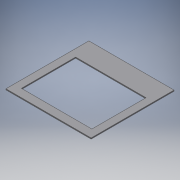
# Autodesk Inventor part: Frontpanel
Saved by Autodesk Inventor 2016 (Build 200138000, 138)
## iProperties
Created: 2018-06-19
Part Number: Frontpanel
Material: Generic
Document SubType Name: Modeling
Designer: suku
Density: 1 g/cm^3
Appearance: Default
Author: suku
Autodesk Inventor part; units mm, degrees
ref_plane "YZ Plane" through (0, 0, 0) normal (1, 0, 0) x (0, 1, 0)
ref_plane "XZ Plane" through (0, 0, 0) normal (0, 1, 0) x (-1, 0, 0)
ref_plane "XY Plane" through (0, 0, 0) normal (0, 0, 1) x (1, 0, 0)
sketch "Sketch1" plane through (0, 0, 0) normal (0, 0, 1) x (1, 0, 0)
  line L0 (109.2, 0) -> (109.2, -84) projected
  line L1 (0, -84) -> (0, 0) projected
  line L2 (0, -84) -> (109.2, -84)
  line L3 (109.2, -84) -> (109.2, 0)
  line L4 (109.2, 0) -> (0, 0)
  line L5 (0, 0) -> (0, -84)
  line L6 (-11.4, 31.9489) -> (120.6, 31.9489)
  line L7 (120.6, 31.9489) -> (120.6, -96.5511)
  line L8 (120.6, -96.5511) -> (-11.4, -96.5511)
  line L9 (-11.4, -96.5511) -> (-11.4, 31.9489)
  line L10 (117.1, 20.1989) -> (-7.9, 20.1989)
  line L11 (-7.9, 20.1989) -> (-7.9, -84.8011)
  line L12 (-7.9, -84.8011) -> (117.1, -84.8011)
  line L13 (117.1, -84.8011) -> (117.1, 20.1989)
  line L14 (-7.9, -84.8011) -> (-7.9, -96.5511)
  line L15 (-7.9, 20.1989) -> (-7.9, 31.9489)
  line L16 (109.2, -42) -> (117.1, -42)
  line L17 (0, -42) -> (-7.9, -42)
  line L18 (120.6, -32.3011) -> (117.1, -32.3011)
  line L19 (-7.9, -32.3011) -> (-11.4, -32.3011)
  dimension "d0" = 128.5
  dimension "d1" = 105
  dimension "d3" = 125
  dimension "d4" = 132
  constraints: 36 end point, 6 midpoint, 6 parallel, 6 point on line, 5 perpendicular, 3 collinear, 3 horizontal
  measures "d0" distance between parallel lines of L8 L6
  measures "d1" distance of L10.end L11.end
  measures "d3" distance between parallel lines of L11 L13
  measures "d4" distance between parallel lines of L7 L9
extrude "Extrusion1" add sketch "Sketch1" against normal blind 1.6 contours L4 L1 L17 L11 L10 L13 L16 L0 | L16 L13 L12 L11 L17 L1 L2 L0 | L13 L18 L7 L8 L14 L12 | L13 L10 L15 L6 L7 L18 | L11 L14 L8 L9 L19 | L19 L9 L6 L15 L11
body "Solid1"
